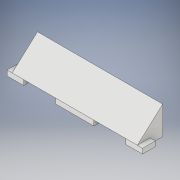
# Autodesk Inventor part: sameSpacer
Saved by Autodesk Inventor 2019 (Build 230136000, 136)
## iProperties
Created: 2020-12-06
Part Number: sameSpacer
Material: Пластик АБС
Document SubType Name: Modeling
Designer: Professional
Density: 1.06 g/cm^3
Appearance: Гладкий — белый
Author: Professional
Autodesk Inventor part; units mm, degrees
ref_plane "YZ Plane" through (0, 0, 0) normal (1, 0, 0) x (0, 1, 0)
ref_plane "XZ Plane" through (0, 0, 0) normal (0, 1, 0) x (-1, 0, 0)
ref_plane "XY Plane" through (0, 0, 0) normal (0, 0, 1) x (1, 0, 0)
sketch "Эскиз1" plane through (0, 0, 0) normal (0, 1, 0) x (-1, 0, 0)
  line L0 (0, 0) -> (10, 0)
  line L1 (10, 0) -> (10, -4)
  line L2 (10, -4) -> (30, -4)
  line L3 (30, -4) -> (30, 0)
  line L4 (30, 0) -> (49, 0)
  line L5 (49, 0) -> (49, 9.8)
  line L6 (49, 9.8) -> (53, 9.8)
  line L7 (53, 9.8) -> (53, 19.8)
  line L8 (53, 19.8) -> (40, 19.8)
  line L9 (40, 19.8) -> (40, 15.8)
  line L10 (40, 15.8) -> (15, 15.8)
  line L11 (15, 15.8) -> (15, 19.8)
  line L12 (15, 19.8) -> (0, 19.8)
  line L13 (0, 19.8) -> (0, 0)
  line L14 (0, 0) -> (-10, 0)
  line L15 (-10, 0) -> (-10, -4)
  line L16 (-10, -4) -> (-30, -4)
  line L17 (-30, -4) -> (-30, 0)
  line L18 (-30, 0) -> (-49, 0)
  line L19 (-49, 0) -> (-49, 9.8)
  line L20 (-49, 9.8) -> (-53, 9.8)
  line L21 (-53, 9.8) -> (-53, 19.8)
  line L22 (-53, 19.8) -> (-40, 19.8)
  line L23 (-40, 19.8) -> (-40, 15.8)
  line L24 (-40, 15.8) -> (-15, 15.8)
  line L25 (-15, 15.8) -> (-15, 19.8)
  line L26 (-15, 19.8) -> (0, 19.8)
  dimension "d0" = 20
  dimension "d1" = 4
  dimension "d2" = 20
  dimension "d3" = 19
  dimension "d4" = 19.8
  dimension "d5" = 30
  dimension "d6" = 25
  dimension "d7" = 10
  constraints: 54 end point, 12 symmetric about line, 11 perpendicular, 8 point on line, 2 equal length, 1 horizontal
  measures "d0" distance of L1.end L2.end
  measures "d1" distance of L2.end L3.end
  measures "d2" diameter of L1 L13
  measures "d3" distance of L3.end L4.end
  measures "d4" distance between parallel lines of L8 L4
  measures "d5" diameter of L11 L13
  measures "d6" distance between parallel lines of L9 L11
  measures "d7" distance between parallel lines of L8 L6
extrude "Выдавливание1" add sketch "Эскиз1" along normal blind 4
sketch "Эскиз2" plane through (0, 4, 0) normal (0, 1, 0) x (1, 0, 0)
  point P0 (0, 0)
sketch "Эскиз3" plane through (49, 0, 9.8) normal (1, 0, 0) x (0, 0, -1)
  line L0 (-10, 4) -> (0, 4) projected
  line L1 (-10, 4) -> (9.8, 22)
  line L2 (9.8, 4) -> (13.8, 4) projected
  line L3 (9.8, 22) -> (9.8, 4)
  line L4 (0, 0) -> (9.8, 0) projected
  line L5 (-10, 4) -> (9.8, 4)
  dimension "d10" = 22
  constraints: 6 end point, 1 collinear, 1 perpendicular
  measures "d10" distance from line of L1.end L4
extrude "Выдавливание2" add sketch "Эскиз3" against normal up to surface (98 mm away)
